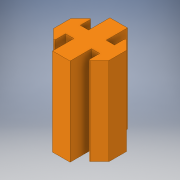
# Autodesk Inventor part: 20X20 lift conecter
Saved by Autodesk Inventor 2019 (Build 230136000, 136)
## iProperties
Created: 2018-10-23
Part Number: 20X20 lift conecter
Material: PC/ABS Plastic
Document SubType Name: Modeling
Designer: User
Density: 0.357273 g/cm^3
Appearance: Orange
Author: User
Autodesk Inventor part; units mm, degrees
ref_plane "YZ Plane" through (0, 0, 0) normal (1, 0, 0) x (0, 1, 0)
ref_plane "XZ Plane" through (0, 0, 0) normal (0, 1, 0) x (-1, 0, 0)
ref_plane "XY Plane" through (0, 0, 0) normal (0, 0, 1) x (1, 0, 0)
sketch "Sketch1" plane through (0, 0, 0) normal (0, 1, 0) x (-1, 0, 0)
  line L0 (0, 0) -> (5.08, 0)
  line L1 (5.08, 0) -> (5.08, -16.637)
  line L2 (5.08, -16.637) -> (0, -16.637)
  line L3 (0, -16.637) -> (0, 0)
  line L4 (0, -6.1892) -> (7.493, -6.1892)
  line L5 (7.493, -6.1892) -> (7.493, -10.4478)
  line L6 (7.493, -10.4478) -> (0, -10.4478)
  line L7 (10.5664, -5.7785) -> (10.5664, -10.8585)
  line L8 (7.493, -13.9319) -> (7.493, -2.7051)
  line L9 (7.493, -13.9319) -> (10.5664, -10.8585)
  line L10 (7.493, -2.7051) -> (10.5664, -5.7785)
  line L11 (0, -6.1892) -> (-2.413, -6.1892)
  line L12 (-2.413, -10.4478) -> (0, -10.4478)
  line L13 (-5.4864, -5.7785) -> (-5.4864, -10.8585)
  line L14 (-2.413, -13.9319) -> (-2.413, -2.7051)
  line L15 (-2.413, -13.9319) -> (-5.4864, -10.8585)
  line L16 (-2.413, -2.7051) -> (-5.4864, -5.7785)
  point P0 (-4.9276, -6.1892)
  dimension "d0" = 5.08
  dimension "d1" = 16.637
  dimension "d2" = 2.413
  dimension "d9" = 3.0734
  dimension "d12" = 0
  dimension "d16" = 11.2268
  dimension "d20" = 135
  dimension "d21" = 135
  dimension "d24" = 6.1893
  dimension "d25" = 16.637
  dimension "d26" = 3.4842
  dimension "d33" = 3.4842
  dimension "d34" = 3.0734
  dimension "d35" = 2.413
  dimension "d36" = 6.1893
  dimension "d37" = 5.08
  dimension "d38" = 5.08
  dimension "d39" = 135
  dimension "d40" = 135
  constraints: 34 end point, 5 point on line, 4 parallel, 2 horizontal, 2 perpendicular
  measures "d0" distance of L1.end L2.end
  measures "d1" distance of L0.end L1.end
  measures "d2" distance between parallel lines of L5 L1
  measures "d9" distance between parallel lines of L7 L8
  measures "d12" distance between parallel lines of L5 L8
  measures "d16" distance of L8.start L8.end
  measures "d20" angle of L9 L7
  measures "d21" angle of L10 L7
  measures "d24" distance between parallel lines of L2 L6
  measures "d25" distance of L2.end L0.start
  measures "d26" distance from line of L4 L8.end
  measures "d33" distance from line of L8.start L12
  measures "d34" distance between parallel lines of L14 L13
  measures "d35" distance between parallel lines of L3 L14
  measures "d36" distance between parallel lines of L0 L4
  measures "d37" distance of L13.start L15.end
  measures "d38" distance of L7.start L7.end
  measures "d39" angle of L13 L15
  measures "d40" angle of L13 L16
extrude "Extrusion2" add sketch "Sketch1" along normal blind 25.4
fillet "Fillet1" radius 0.254 4 edges at (2.413, 12.7, -13.9319) (-7.493, 12.7, -13.9319) (2.413, 12.7, -2.7051) (-7.493, 12.7, -2.7051)
equation "\"d16\" = d15"
equation "\"d21\" = d20"
equation "\"d24\" = -0.5 * d4 + 0.5 * d25"
equation "\"d15\" = 11.2268"
equation "\"d4\" = 4.2585"
body "Solid2"
